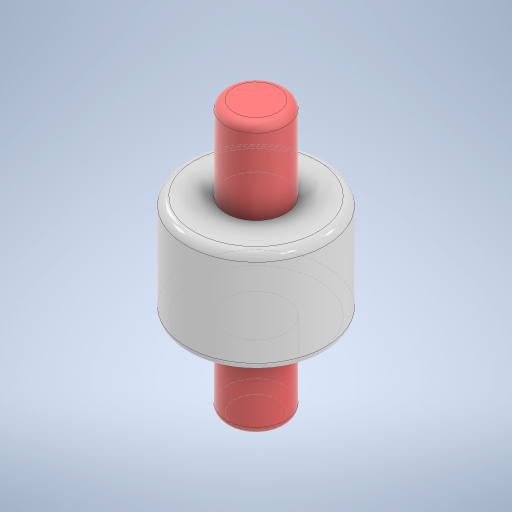
# Autodesk Inventor part: Amostra_v1
Saved by Autodesk Inventor 2024 (Build 280153000, 153)
## iProperties
Created: 2025-07-22
Part Number: Amostra_v1
Material: Generic
Document SubType Name: Modeling
Designer: Bruno
Density: 1 g/cm^3
Appearance: Default
Author: Bruno
Autodesk Inventor part; units mm, degrees
ref_plane "YZ Plane" through (0, 0, 0) normal (1, 0, 0) x (0, 1, 0)
ref_plane "XZ Plane" through (0, 0, 0) normal (0, 1, 0) x (-1, 0, 0)
ref_plane "XY Plane" through (0, 0, 0) normal (0, 0, 1) x (1, 0, 0)
sketch "Sketch1" plane through (0, 0, 0) normal (0, 1, 0) x (-1, 0, 0)
  circle A0 centre (0, 0) radius 17.5
  circle A1 centre (0, 0) radius 7.5
  dimension "d0" = 35
  dimension "d1" = 15
  constraints: 2 centre point, 2 coincident
  measures "d0" diameter of A0
  measures "d1" diameter of A1
extrude "Extrusion1" add sketch "Sketch1" along normal blind 26
sketch "Sketch2" plane through (0, 0, 0) normal (0, -1, 0) x (1, 0, 0)
  circle A0 centre (0, 0) radius 7.5 projected
extrude "Extrusion2" add sketch "Sketch2" along normal blind 21 and the other way blind 47
fillet "Fillet1" radius 2 4 edges at (17.5, 26, 0) (17.5, 0, 0) (-7.5, 47, 0) (-7.5, -21, 0)
body "Solid1"
